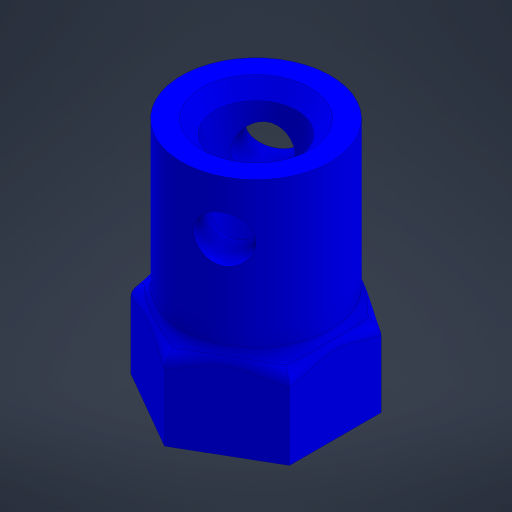
# Autodesk Inventor part: hex
Saved by Autodesk Inventor 2024 (Build 280153000, 153)
## iProperties
Created: 2023-11-15
Part Number: hex
Material: Типовые
Document SubType Name: Modeling
Designer: user
Density: 1 g/cm^3
Appearance: По умолчанию
Author: user
Autodesk Inventor part; units mm, degrees
ref_plane "YZ Plane" through (0, 0, 0) normal (1, 0, 0) x (0, 1, 0)
ref_plane "XZ Plane" through (0, 0, 0) normal (0, 1, 0) x (-1, 0, 0)
ref_plane "XY Plane" through (0, 0, 0) normal (0, 0, 1) x (1, 0, 0)
sketch "Эскиз1" plane through (0, 0, 0) normal (0, 0, 1) x (1, 0, 0)
  circle A0 centre (0, 0) radius 5.65
  circle A1 centre (0, 0) radius 3.1
  dimension "d0" = 6.2
  dimension "d1" = 11.3
  constraints: 2 centre point, 2 coincident
  measures "d0" diameter of A1
  measures "d1" diameter of A0
extrude "Выдавливание1" add sketch "Эскиз1" against normal blind 12
sketch "Эскиз2" plane through (0, 0, -12) normal (0, 0, -1) x (-1, 0, 0)
  circle A0 centre (0, 0) radius 3.1 construction
  line L0 (6, 3.4641) -> (6, -3.4641)
  line L1 (6, -3.4641) -> (0, -6.9282)
  line L2 (0, -6.9282) -> (-6, -3.4641)
  line L3 (-6, -3.4641) -> (-6, 3.4641)
  line L4 (-6, 3.4641) -> (0, 6.9282)
  line L5 (0, 6.9282) -> (6, 3.4641)
  circle A1 centre (0, 0) radius 2
  dimension "d4" = 12
  dimension "d5" = 4
  constraints: 12 end point, 2 coincident, 1 centre point, 1 vertical, 13 other
  measures "d4" distance of L3.end L0.start
  measures "d5" diameter of A1
extrude "Выдавливание2" add sketch "Эскиз2" along normal blind 6
chamfer "Фаска1" distance 1 angle 45 1 edges at (-3.1, 0, 0)
fillet "Сопряжение1" radius 1 7 edges at (-5.65, 0, -12) (6, 0, -12) (3, -5.1962, -12) (3, 5.1962, -12) (-3, 5.1962, -12) (-6, 0, -12) (-3, -5.1962, -12)
sketch "Эскиз3" plane through (0, -6.9282, -18) normal (0.5, -0.8660254, 0) x (0.8660254, 0.5, 0)
  circle A0 centre (3.1757, 13.9) radius 1.7489
  point P0 (3.4641, 18)
  dimension "d12" = 4.1
  constraints: 1 centre point
  measures "d12" vertical distance of point (3.464, 18) A0.centre
extrude "Выдавливание3" cut sketch "Эскиз3" against normal through all
